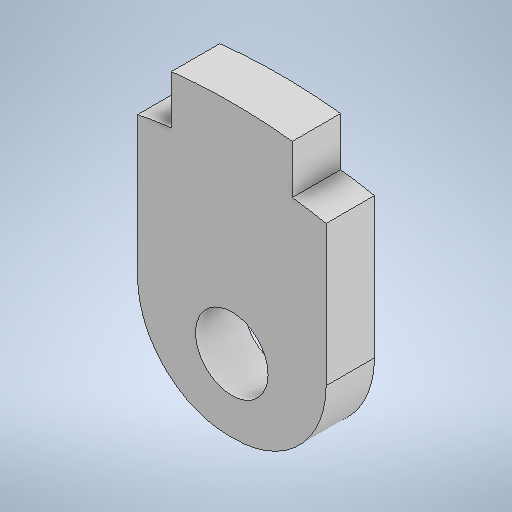
# Autodesk Inventor part: ModuleConnector_Outside_Axis
Saved by Autodesk Inventor 2025.1 (Build 291241020, 241B)
## iProperties
Created: 2024-10-09
Part Number: ModuleConnector_Outside_Axis
Material: 일반
Document SubType Name: Modeling
Designer: SEON06
Density: 1 g/cm^3
Appearance: 기본값
Author: SEON06
## iProperties of the stored document ModuleConnector_Outside_Axis_3D 인쇄.ipt
Created: 2024-10-12
Part Number: ModuleConnector_Outside_Axis_3D 인쇄
Material: 일반
Document SubType Name: Modeling
Designer: SEON06
Density: 1 g/cm^3
Appearance: 기본값
Author: SEON06
Autodesk Inventor part; units mm, degrees
ref_plane "YZ Plane" through (0, 0, 0) normal (1, 0, 0) x (0, 1, 0)
ref_plane "XZ Plane" through (0, 0, 0) normal (0, 1, 0) x (-1, 0, 0)
ref_plane "XY Plane" through (0, 0, 0) normal (0, 0, 1) x (1, 0, 0)
sketch "스케치1" plane through (0, 0, 0) normal (0, 0, 1) x (1, 0, 0)
  circle A0 centre (0, 0) radius 20
  line L0 (-3.9, 19.6161) -> (-3.9, 0)
  line L1 (-3.9, 0) -> (3.9, 0)
  line L2 (3.9, 0) -> (3.9, 19.6161)
  circle A1 centre (0, 0) radius 10
  line L3 (-2.5, 21.8575) -> (-2.5, 19.8431)
  line L4 (2.5, 21.8575) -> (2.5, 19.8431)
  circle A2 centre (0, 0) radius 22
  point P0 (0, 0)
  point P1 (0, 0)
  point P2 (-3.9, 9.2081)
  point P3 (3.9, 9.2081)
  dimension "d0" = 40
  dimension "d1" = 7.8
  dimension "d5" = 20
  dimension "d13" = 2
  dimension "d14" = 5
  dimension "d15" = 2.5
  constraints: 10 end point, 6 point on circle, 5 coincident, 3 centre point, 3 vertical, 2 perpendicular, 1 midpoint
  measures "d0" diameter of A0
  measures "d1" distance of L0.end L1.end
  measures "d5" diameter of A1
  measures "d13" radial gap between concentric circles of A0 A2
  measures "d14" distance between parallel lines of L4 L3
  measures "d15" distance from line of point (0, 0) L3
extrude "돌출1" add sketch "스케치1" along normal blind 2 contours L2 A1 L0 A0 | A0 L3 A2 L4 picked at (1.4966, 13.2144) picked at (-1.9451, 20.5611)
sketch "스케치2" plane through (0, 0, 2) normal (0, 0, 1) x (1, 0, 0)
  circle A0 centre (0, 13) radius 1.5
  arc A1 (3.9, 9.2081) -> (-3.9, 9.2081) centre (0, 0) ccw projected
  point P0 (0, 0)
  point P1 (0, 10)
  dimension "d6" = 3
  dimension "d7" = 3
  constraints: 1 centre point, 1 point on circle, 1 vertical alignment
  measures "d6" diameter of A0
  measures "d7" distance of point (0, 10) A0.centre
extrude "돌출2" cut sketch "스케치2" against normal through all
fillet "모깎기1" radius 3.8 2 edges at (-3.9, 9.2081, 1) (3.9, 9.2081, 1)
equation "\"d15\" = 0.5 * d14"
